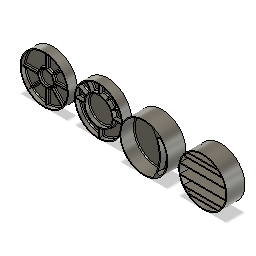
parts-tray1 (Autodesk Fusion 360 design; units mm, degrees)
Autodesk Fusion 360 part; units mm, degrees
sketch "Sketch1" plane through (0, 0, 0) normal (0, 0, 1) x (1, 0, 0) in component "parts-tray"
  circle A0 centre (0, 0) radius 26.5
  dimension "d1" = 53
  constraint coincident A0.centre origin
  measures "d1" diameter of A0
extrude "Extrude1" add sketch "Sketch1" along normal blind 10 contours A0 picked at (-3.934332, 6.420922) makes body 1 in component "parts-tray"
sketch "Sketch2" plane through (0, 0, 10) normal (0, 0, 1) x (1, 0, 0) in component "parts-tray"
  circle A0 centre (0, 0) radius 26.5
  circle A1 centre (0, 0) radius 15
  line L0 (0.5, -25.870951) -> (-0.5, 25.870951) construction
  line L1 (-0.5, -25.870951) -> (0.5, 25.870951) construction
  line L2 (26.077284, -0.5) -> (-26.077284, 0.5) construction
  line L3 (-26.077284, -0.5) -> (26.077284, 0.5) construction
  line L4 (15.992186, 0.5) -> (26.077284, 0.5)
  line L5 (26.077284, -0.5) -> (15.992186, -0.5)
  line L6 (-26.077284, 0.5) -> (-15.992186, 0.5)
  line L7 (0.5, 25.870951) -> (0.5, 15.992186)
  line L8 (-0.5, 15.992186) -> (-0.5, 25.870951)
  line L9 (-0.5, -25.870951) -> (-0.5, -15.992186)
  line L10 (0.5, -15.992186) -> (0.5, -25.870951)
  line L11 (0.5, -0.5) -> (-14.991664, -0.5)
  line L12 (-15.992186, -0.5) -> (-26.077284, -0.5)
  arc A2 (-15.99706, -0.306724) -> (-0.309169, -15.997013) centre (0, 0) ccw
  arc A3 (0.309169, -15.997013) -> (15.99706, -0.306724) centre (0, 0) ccw
  arc A4 (-25.495314, -0.488841) -> (-0.492739, -25.495239) centre (0, 0) ccw
  arc A5 (0.492739, -25.495239) -> (25.495314, -0.488841) centre (0, 0) ccw
  line L13 (0, 0) -> (25.833701, 0) construction
  line L14 (0, 0) -> (25.728452, 0) construction
  line L15 (0, 0) -> (25.997652, 0) construction
  line L16 (0, 0) -> (25.798155, 0) construction
  line L17 (0, 0) -> (25.810188, 0) construction
  line L18 (0, 0) -> (25.861248, 0) construction
  line L19 (0, 0) -> (25.942244, 0) construction
  arc A6 (-22.720666, 11.576758) -> (-25.495314, 0.488841) centre (0, 0) ccw
  arc A7 (-0.492739, 25.495239) -> (-12.75, 22.083648) centre (0, 0) ccw
  arc A8 (-13.888295, 21.386099) -> (-22.083648, 12.75) centre (0, 0) ccw
  arc A9 (12.75, 22.083648) -> (0.492739, 25.495239) centre (0, 0) ccw
  arc A10 (25.495314, 0.488841) -> (22.720666, 11.576758) centre (0, 0) ccw
  arc A11 (22.083648, 12.75) -> (13.888295, 21.386099) centre (0, 0) ccw
  line L20 (14.256104, 7.263848) -> (23.16617, 11.803753)
  line L21 (22.372642, 12.916851) -> (13.856406, 8)
  line L22 (8.714225, 13.418729) -> (14.159336, 21.803465)
  line L23 (8, 13.856406) -> (12.864226, 22.281493)
  line L24 (-8, 13.856406) -> (-12.899078, 22.341858)
  line L25 (-8.714225, 13.418729) -> (-14.057236, 21.646245)
  line L26 (-13.856406, 8) -> (-22.396498, 12.930624)
  line L27 (-14.256104, 7.263848) -> (-23.114709, 11.777532)
  arc A12 (-14.256104, 7.263848) -> (-15.99706, 0.306724) centre (0, 0) ccw
  arc A13 (-0.309169, 15.997013) -> (-8, 13.856406) centre (0, 0) ccw
  arc A14 (-8.714225, 13.418729) -> (-13.856406, 8) centre (0, 0) ccw
  arc A15 (8, 13.856406) -> (0.309169, 15.997013) centre (0, 0) ccw
  line L28 (13.856406, 8) -> (22.372642, 12.916851)
  arc A16 (15.99706, 0.306724) -> (14.256104, 7.263848) centre (0, 0) ccw
  arc A17 (13.856406, 8) -> (8.714225, 13.418729) centre (0, 0) ccw
  dimension "d4" = 51
  dimension "d5" = 30
  dimension "d6" = 32
  dimension "d7" = 1
  dimension "d8" = 1
  dimension "d11" = 26
  constraint coincident A0.centre A1.centre
  constraint parallel L7 L9
  constraint horizontal L5
  constraint parallel L5 L6
  constraint collinear L4 L6
  constraint collinear L5 L11
  constraint coincident L11.start L7
  constraint collinear L8 L9
  constraint collinear L11 L12
  constraint horizontal L13
  constraint horizontal L14
  constraint horizontal L15
  constraint horizontal L16
  constraint horizontal L17
  constraint horizontal L18
  constraint horizontal L19
  measures "d4" diameter of A7
  measures "d5" diameter of A1
  measures "d6" diameter of A16
extrude "Extrude2" cut sketch "Sketch2" against normal blind 5 contours A1 | L4 A10 L20 A16 | L5 L10 A3 A5 | L6 A6 L27 A12 | L7 A9 L23 A15 | L8 A7 L24 A13 | L9 L12 A2 A4 | A8 L25 L26 A14 | A11 L21 L22 L28 A17 picked at (-4.327629, 3.139882) picked at (21.919913, 4.132211) picked at (1.677832, -22.222087) picked at (-21.919913, 4.132211) picked at (1.56662, 22.239148) picked at (-1.56662, 22.239148) picked at (-22.222087, -1.677832) picked at (-15.011255, 16.486659) picked at (15.011255, 16.486659) bodies 1 in component "parts-tray"
fillet "Fillet1" radius 1 33 edges at (-18.031223, -18.031223, 5) (-20.743642, -0.5, 5) (11.313708, -11.313708, 5) (20.743642, -0.5, 5) (18.488385, 9.420303, 5) (15.497651, 3.977792, 5) (11.30126, 17.402414, 5) (18.497046, 17.553042, 5) (6.841061, 24.565217, 5) (0.5, 20.743642, 5) (-6.841061, 24.565217, 5) (-10.375, 17.970027, 5) (-18.497046, 17.553042, 5) (-18.488385, 9.420303, 5) (-24.735877, 6.195675, 5) (-4.38211, 15.388213, 5) (-17.970027, 10.375, 5) (4.38211, 15.388213, 5) (-13.98491, 5.424231, 5) (11.60599, 11.013673, 5) (17.970027, 10.375, 5) (-20.743642, 0.5, 5) (0.5, -20.743642, 5) (18.031223, -18.031223, 5) (20.743642, 0.5, 5) (24.735877, 6.195675, 5) (-0.5, -20.743642, 5) (-15.497651, 3.977792, 5) (-11.60599, 11.013673, 5) (-11.30126, 17.402414, 5) (10.375, 17.970027, 5) (-0.5, 20.743642, 5) (-11.313708, -11.313708, 5) on bodies 1 in component "parts-tray"
sketch "Sketch1 (2)" plane through (0, 0, 0) normal (0, 0, -1) x (-1, 0, 0) in component "parts-tray2"
  circle A0 centre (0, 0) radius 26.5
  circle A1 centre (0, 0) radius 26.5
  constraint coincident A0.centre A1.centre
extrude "Extrude1'" add sketch "Sketch1 (2)" against normal blind 20 separate body contours A0 A1 picked at (-3.934332, 6.420922) makes body 2 in component "parts-tray2"
sketch "Sketch2 (2)" plane through (0, 0, 20) normal (0, 0, 1) x (1, 0, 0) in component "parts-tray2"
  circle A0 centre (0, 0) radius 26.5
  circle A1 centre (0, 0) radius 25.5
  arc A2 (10.022742, -23.4477) -> (9.956675, 23.475831) centre (-25.765763, -0.036278) ccw
  arc A3 (15.257312, -15.670904) -> (15.218991, 15.572451) centre (-25.191842, -0.098815) ccw
  arc A4 (18.150921, 17.910725) -> (15.218991, 15.572451) centre (17.050822, 16.282833) ccw
  arc A5 (15.257312, -15.670904) -> (18.482872, -17.567966) centre (17.027215, -16.35228) ccw
  dimension "d24" = 51
  constraint coincident A0.centre A1.centre
  constraint tangent A2 A3
  constraint tangent A3 A4
  constraint tangent A3 A5
  measures "d24" diameter of A1
extrude "Extrude2'" cut sketch "Sketch2 (2)" against normal blind 15 contours A1 A2 picked at (3.251806, -5.09518) bodies 2 in component "parts-tray2"
extrude "Extrude3" cut sketch "Sketch2 (2)" against normal blind 8 contours A1 A3 A4 A5 picked at (20.522282, -0.030532) bodies 2 in component "parts-tray2"
fillet "Fillet1'" radius 1 4 edges at (15.954753, -17.916459, 12) (18.151222, -0.045653, 12) (15.825775, 17.818903, 12) (25.499775, 0.107115, 12) on bodies 2 in component "parts-tray2"
fillet "Fillet2" radius 1 2 edges at (16.999973, 0.023936, 5) (-25.499975, -0.035903, 5) on bodies 2 in component "parts-tray2"
sketch "Sketch2 (3)" plane through (0, 0, 5) normal (0, 0, 1) x (1, 0, 0) in component "parts-tray3"
  circle A0 centre (0, 0) radius 14
  circle A1 centre (-75, 0) radius 26.5
  circle A2 centre (-75, 0) radius 25.5
  line L0 (-75.500001, 8.299322) -> (-75.500001, 25.700679)
  line L1 (-74.500001, 25.700679) -> (-74.500001, 8.299322)
  line L2 (-74.500001, 8.299322) -> (-75.500001, 25.700679) construction
  line L3 (-75.500001, 8.299322) -> (-74.500001, 25.700679) construction
  line L4 (-69.485047, 6.222061) -> (-57.18043, 18.526678)
  line L5 (-56.473323, 17.819571) -> (-68.777941, 5.514954)
  line L6 (-66.700678, 0.500001) -> (-49.299321, 0.500001)
  line L7 (-49.299321, -0.499999) -> (-66.700678, -0.499999)
  line L8 (-68.777939, -5.514953) -> (-56.473322, -17.81957)
  line L9 (-57.180429, -18.526677) -> (-69.485046, -6.222059)
  line L10 (-74.499999, -8.299322) -> (-74.499999, -25.700679)
  line L11 (-75.499999, -25.700679) -> (-75.499999, -8.299322)
  line L12 (-80.514953, -6.222061) -> (-92.81957, -18.526678)
  line L13 (-93.526677, -17.819571) -> (-81.222059, -5.514954)
  line L14 (-83.299322, -0.500001) -> (-100.700679, -0.500001)
  line L15 (-100.700679, 0.499999) -> (-83.299322, 0.499999)
  circle A3 centre (-75, 0) radius 8
  arc A4 (-68.999422, 6.707687) -> (-74.53959, 8.988216) centre (-75, 0) ccw
  arc A5 (-66.0139, 0.500001) -> (-68.292315, 6.00058) centre (-75, 0) ccw
  arc A6 (-68.292313, -6.000578) -> (-66.013899, -0.499999) centre (-75, 0) ccw
  arc A7 (-74.499999, -8.9861) -> (-68.99942, -6.707685) centre (-75, 0) ccw
  arc A8 (-81.000578, -6.707687) -> (-75.499999, -8.986101) centre (-75, 0) ccw
  arc A9 (-75.460413, 8.988216) -> (-83.986101, 0.499999) centre (-75, 0) ccw
  arc A10 (-83.9861, -0.500001) -> (-81.707685, -6.00058) centre (-75, 0) ccw
  point P0 (-75.000001, 17)
  dimension "d33" = 53
  dimension "d34" = 51
  dimension "d35" = 1
  dimension "d36" = 1
  dimension "d37" = 1
  dimension "d38" = 1
  dimension "d39" = 1
  dimension "d40" = 1
  dimension "d41" = 1
  dimension "d42" = 18
  constraint concentric A1 A2
  constraint parallel L0 L1
  constraint parallel L4 L5
  constraint parallel L6 L7
  constraint parallel L8 L9
  constraint parallel L10 L11
  constraint parallel L12 L13
  constraint parallel L14 L15
  constraint concentric A1 A3
  constraint concentric A1 A9
  constraint concentric A4 A9
  constraint concentric A5 A9
  constraint concentric A6 A9
  constraint concentric A7 A9
  constraint concentric A8 A9
  constraint concentric A9 A10
  measures "d33" diameter of A1
  measures "d34" diameter of A2
  measures "d42" diameter of A9
extrude "Extrude1''" add sketch "Sketch2 (3)" against normal blind 10 separate body contours A1 | A2 L0 L1 L4 L5 L6 L7 L8 L9 L10 L11 L12 L13 L14 L15 A4 A5 A6 A7 A8 A9 A10 | A2 L5 L6 A5 | A2 L7 L8 A6 | A2 L1 L4 A4 | A2 L9 L10 A7 | A2 L0 L15 A9 | A2 L11 L12 A8 | A2 L13 L14 A10 | A3 picked at (-91.313818, -19.968231) picked at (-60.509266, 0.000001) picked at (-55.127142, 1.761708) picked at (-59.702051, -12.806517) picked at (-62.193483, 15.297949) picked at (-73.238292, -19.872858) picked at (-89.113018, 14.113017) picked at (-87.806517, -15.297949) picked at (-94.872858, -1.761708) picked at (-75.19928, 2.540405) makes body 3 in component "parts-tray3"
extrude "Extrude2''" cut sketch "Sketch2 (3)" against normal blind 5 contours A2 L5 L6 A5 | A2 L7 L8 A6 | A2 L1 L4 A4 | A2 L9 L10 A7 | A2 L0 L15 A9 | A2 L11 L12 A8 | A2 L13 L14 A10 | A3 picked at (-55.127142, 1.761708) picked at (-59.702051, -12.806517) picked at (-62.193483, 15.297949) picked at (-73.238292, -19.872858) picked at (-89.113018, 14.113017) picked at (-87.806517, -15.297949) picked at (-94.872858, -1.761708) picked at (-75.19928, 2.540405) bodies 3 in component "parts-tray3"
extrude "Extrude3'" cut sketch "Sketch2 (3)" against normal blind 2 contours A2 L0 L1 L4 L5 L6 L7 L8 L9 L10 L11 L12 L13 L14 L15 A4 A5 A6 A7 A8 A9 A10 picked at (-60.509266, 0.000001) bodies 3 in component "parts-tray3"
fillet "Fillet1''" radius 1 8 faces at (-89.113018, 14.113017, 0) (-62.193483, 15.297949, 0) (-55.127142, 1.761708, 0) (-75.19928, 2.540405, 0) (-73.238292, -19.872858, 0) (-87.806517, -15.297949, 0) (-94.872858, -1.761708, 0) (-59.702051, -12.806517, 0) on bodies 3 in component "parts-tray3"
sketch "Sketch1 (3)" plane through (0, 0, 0) normal (0, 0, 1) x (1, 0, 0) in component "parts-tray4"
  circle A0 centre (125, 0) radius 26.5
  dimension "d51" = 53
  measures "d51" diameter of A0
extrude "Extrude1'''" add sketch "Sketch1 (3)" along normal blind 20 separate body contours A0 picked at (128.227179, 8.222718) makes body 4 in component "parts-tray4"
sketch "Sketch2 (4)" plane through (0, 0, 20) normal (0, 0, 1) x (1, 0, 0) in component "parts-tray4"
  circle A0 centre (125, 0) radius 26.5
  circle A1 centre (125, 0) radius 25.5
  line L0 (150.005, 5) -> (99.995, 5)
  line L1 (150.684954, 5) -> (99.315046, -5) construction
  line L2 (99.969849, 4.872532) -> (150.684954, -5) construction
  line L3 (154.269779, 6) -> (95.730221, -6) construction
  line L4 (95.730221, 6) -> (154.269779, -6) construction
  line L5 (95.000001, 6) -> (95.000001, 14)
  line L6 (154.269779, 14) -> (154.269779, 6)
  line L7 (95.000001, 14) -> (146.313141, 14)
  line L8 (154.269779, 14) -> (154.269779, 15)
  line L9 (145.621591, 15) -> (95.000001, 15)
  line L10 (95.000001, 15) -> (95.000001, 14)
  line L11 (145.621591, 15) -> (95.000001, 15)
  line L12 (95.000001, 15) -> (95.000001, 19)
  line L13 (154.269779, 19) -> (154.269779, 15)
  line L14 (154.405055, 19) -> (154.405055, 20)
  line L15 (140.819292, 20) -> (109.180708, 20)
  line L16 (95.000001, 20) -> (95.000001, 19)
  line L17 (107.992649, 19) -> (142.007351, 19)
  line L18 (107.992649, 19) -> (142.007351, 19)
  line L19 (154.269779, 19) -> (154.405055, 19)
  line L20 (95.000001, 14) -> (146.313141, 14)
  line L21 (149.784067, 6) -> (100.215933, 6)
  line L22 (149.784067, 6) -> (100.215933, 6)
  line L23 (95.730221, 6) -> (95.000001, 6)
  line L24 (99.995, -5) -> (150.005, -5)
  line L25 (100.215933, -6) -> (149.784067, -6)
  line L26 (154.999999, -14) -> (103.686859, -14)
  line L27 (104.378409, -15) -> (154.999999, -15)
  line L28 (142.007351, -19) -> (107.992649, -19)
  line L29 (109.180708, -20) -> (140.819292, -20)
  point P0 (125, 0)
  point P1 (125, 0)
  dimension "d54" = 51
  dimension "d56" = 12
  dimension "d57" = 8
  dimension "d58" = 1
  dimension "d59" = 4
  dimension "d60" = 1
  constraint concentric A0 A1
  constraint horizontal L0
  constraint coincident L1 P1
  constraint coincident L2 P1
  constraint coincident P1 P0
  constraint coincident L3 P1
  constraint coincident L4 P1
  constraint horizontal L22
  constraint vertical L5
  constraint horizontal L20
  constraint vertical L6
  constraint horizontal L7
  constraint vertical L8
  constraint horizontal L9
  constraint vertical L10
  constraint horizontal L11
  constraint vertical L12
  constraint vertical L13
  constraint horizontal L18
  constraint vertical L14
  constraint horizontal L15
  constraint vertical L16
  constraint collinear L18 L19
  constraint collinear L22 L23
  constraint coincident A1 L0.end
  constraint coincident A1 L0.start
  measures "d54" diameter of A1
extrude "Extrude2'''" cut sketch "Sketch2 (4)" against normal blind 19 contours A1 L9 L11 L17 L18 | A1 L25 L26 | A1 L7 L20 L21 L22 | A1 L27 L28 | A1 L0 L24 picked at (118.126136, 17.666667) picked at (117.89562, -8.666667) picked at (117.408756, 7.824005) picked at (131.873864, -17.666667) picked at (133.481614, -0.558775) bodies 4 in component "parts-tray4"
extrude "Extrude3''" cut sketch "Sketch2 (4)" against normal blind 15 contours A1 L15 | A1 L29 picked at (129.133816, 21.960333) picked at (129.227128, -20.707707) bodies 4 in component "parts-tray4"
fillet "Fillet1'''" radius 1 7 faces at (129.133816, 21.960333, 5) (118.126136, 17.666667, 1) (117.408756, 7.824005, 1) (133.335, -1.666667, 1) (117.89562, -8.666667, 1) (131.873864, -17.666667, 1) (129.227128, -20.707707, 5) on bodies 4 in component "parts-tray4"
component "parts-tray" placed x (1, 0, 0) y (0, 1, 0) z (0, 0, 1) at (0, 0, 0)
component "parts-tray2" placed x (1, 0, 0) y (0, 1, 0) z (0, 0, 1) at (60, 0, 0)
component "parts-tray3" placed x (1, 0, 0) y (0, 1, 0) z (0, 0, 1) at (15, 0, 5)
component "parts-tray4" placed x (1, 0, 0) y (0, 1, 0) z (0, 0, 1) at (0, 0, 0)
